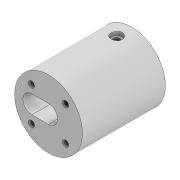
# Autodesk Inventor part: Part1_b_nmew
Saved by Autodesk Inventor 2021 (Build 250183000, 183)
## iProperties
Created: 2022-05-23
Part Number: Part1_b_nmew
Material: Generic
Document SubType Name: Modeling
Designer: romanp
Density: 1 g/cm^3
Appearance: Default
Author: romanp
Autodesk Inventor part; units mm, degrees
ref_plane "YZ Plane" through (0, 0, 0) normal (1, 0, 0) x (0, 1, 0)
ref_plane "XZ Plane" through (0, 0, 0) normal (0, 1, 0) x (-1, 0, 0)
ref_plane "XY Plane" through (0, 0, 0) normal (0, 0, 1) x (1, 0, 0)
sketch "Sketch11" plane through (0, 0, 0) normal (0, 0, 1) x (1, 0, 0)
  line L0 (-3.4593, 3.4593) -> (0, 0)
  line L1 (-3.4593, 3.4593) -> (-3.4593, 46.5407)
  line L2 (0, 50) -> (-3.4593, 46.5407)
  line L3 (43.0814, 50) -> (0, 50)
  line L4 (46.5407, 46.5407) -> (43.0814, 50)
  line L5 (46.5407, 3.4593) -> (46.5407, 46.5407)
  line L6 (43.0814, 0) -> (46.5407, 3.4593)
  line L7 (43.0814, 0) -> (0, 0)
  constraints: 16 end point
extrude "Extrusion8" add sketch "Sketch11" along normal blind 5
sketch "Sketch16" plane through (0, 0, 0) normal (0, 0, -1) x (-1, 0, 0)
  line L0 (-27.0407, 40) -> (-34.0407, 40)
  line L1 (-36.5407, 37.5) -> (-36.5407, 30.5)
  arc A0 (-34.0407, 40) -> (-36.5407, 37.5) centre (-34.0407, 37.5) ccw
  line L2 (-9.0407, 40) -> (-16.0407, 40)
  arc A1 (-6.5407, 37.5) -> (-9.0407, 40) centre (-9.0407, 37.5) ccw
  line L3 (-6.5407, 30.5) -> (-6.5407, 37.5)
  line L4 (-6.5407, 12.5) -> (-6.5407, 19.5)
  arc A2 (-9.0407, 10) -> (-6.5407, 12.5) centre (-9.0407, 12.5) ccw
  line L5 (-16.0407, 10) -> (-9.0407, 10)
  line L6 (-34.0407, 10) -> (-27.0407, 10)
  arc A3 (-36.5407, 12.5) -> (-34.0407, 10) centre (-34.0407, 12.5) ccw
  line L7 (-36.5407, 19.5) -> (-36.5407, 12.5)
  line L8 (0, 50) -> (3.4593, 46.5407) projected
  line L9 (-43.0814, 0) -> (-46.5407, 3.4593) projected
  line L10 (-46.5407, 46.5407) -> (-43.0814, 50) projected
  line L11 (-43.0814, 0) -> (-43.0814, 50)
  line L12 (3.4593, 3.4593) -> (0, 0) projected
  line L13 (-6.5407, 30.5) -> (-6.5407, 19.5)
  line L14 (-16.0407, 40) -> (-27.0407, 40)
  line L15 (-36.5407, 30.5) -> (-36.5407, 19.5)
  line L16 (-27.0407, 10) -> (-16.0407, 10)
  circle A4 centre (-2.5407, 44) radius 2.5
  circle A5 centre (-40.5407, 6) radius 2.5
  circle A6 centre (-2.5407, 6) radius 2.5
  circle A7 centre (-40.5407, 44) radius 2.5
  line L17 (0, 50) -> (3.4593, 46.5407)
  line L18 (3.4593, 46.5407) -> (3.4593, 3.4593) projected
  line L19 (0, 0) -> (-43.0814, 0) projected
  line L20 (3.4593, 3.4593) -> (0, 0)
  line L21 (0, 0) -> (-43.0814, 0)
  line L22 (-43.0814, 0) -> (-46.5407, 3.4593) projected
  line L23 (-43.0814, 0) -> (-46.5407, 3.4593)
  line L24 (-46.5407, 3.4593) -> (-46.5407, 46.5407) projected
  line L25 (-46.5407, 3.4593) -> (-46.5407, 46.5407)
  line L26 (-46.5407, 46.5407) -> (-43.0814, 50)
  line L27 (0, 50) -> (-43.0814, 50) projected
  line L28 (0, 50) -> (-43.0814, 50)
  dimension "d44" = 5
  dimension "d45" = 5
  dimension "d46" = 5
  dimension "d47" = 5
  constraints: 40 end point, 8 centre point, 8 collinear, 8 point on circle, 2 vertical, 1 perpendicular, 1 point on line
  measures "d44" diameter of A4
  measures "d45" diameter of A5
  measures "d46" diameter of A6
  measures "d47" diameter of A7
extrude "Extrusion11" add sketch "Sketch16" along normal blind 15
sketch "Sketch18" plane through (0, 0, -15) normal (0, 0, -1) x (-1, 0, 0)
  circle A0 centre (-2.5407, 6) radius 2.5 projected
  circle A1 centre (-2.5407, 6) radius 2.5
  circle A2 centre (-40.5407, 6) radius 2.5 projected
  circle A3 centre (-40.5407, 6) radius 2.5
  circle A4 centre (-40.5407, 44) radius 2.5 projected
  circle A5 centre (-40.5407, 44) radius 2.5
  circle A6 centre (-2.5407, 44) radius 2.5 projected
  circle A7 centre (-2.5407, 44) radius 2.5
  point P0 (0, 0)
  constraints: 4 centre point, 4 coincident
extrude "Extrusion12" cut sketch "Sketch18" against normal blind 100
sketch "Sketch19" plane through (0, 0, -15) normal (0, 0, -1) x (-1, 0, 0)
  circle A0 centre (-2.5407, 6) radius 2.5 projected
  circle A1 centre (-2.5407, 6) radius 4.3
  circle A2 centre (-40.5407, 6) radius 2.5 projected
  circle A3 centre (-40.5407, 6) radius 4.3
  circle A4 centre (-2.5407, 44) radius 2.5 projected
  circle A5 centre (-2.5407, 44) radius 4.3
  circle A6 centre (-40.5407, 44) radius 2.5 projected
  circle A7 centre (-40.5407, 44) radius 4.3
  point P0 (0, 0)
  dimension "d54" = 8.6
  dimension "d55" = 8.6
  dimension "d56" = 8.6
  dimension "d57" = 8.6
  constraints: 4 centre point, 4 coincident
  measures "d54" diameter of A1
  measures "d55" diameter of A3
  measures "d56" diameter of A5
  measures "d57" diameter of A7
extrude "Extrusion13" cut sketch "Sketch19" against normal blind 10 contours A0 | A1 | A2 | A3 | A5 | A6 | A7
sketch "Sketch20" plane through (0, 0, -15) normal (0, 0, -1) x (-1, 0, 0)
  line L0 (0, 50) -> (-43.0814, 50) projected
  line L1 (-43.0814, 50) -> (-46.5407, 46.5407) projected
  line L2 (-46.5407, 46.5407) -> (-46.5407, 3.4593) projected
  line L3 (-46.5407, 3.4593) -> (-43.0814, 0) projected
  line L4 (-43.0814, 0) -> (0, 0) projected
  line L5 (0, 0) -> (3.4593, 3.4593) projected
  line L6 (3.4593, 3.4593) -> (3.4593, 46.5407) projected
  line L7 (3.4593, 46.5407) -> (0, 50) projected
  circle A0 centre (-2.5407, 44) radius 4.3 projected
  circle A1 centre (-40.5407, 44) radius 4.3 projected
  circle A2 centre (-40.5407, 6) radius 4.3 projected
  circle A3 centre (-2.5407, 6) radius 4.3 projected
  arc A4 (-9.0407, 10) -> (-6.5407, 12.5) centre (-9.0407, 12.5) ccw projected
  line L8 (-9.0407, 10) -> (-34.0407, 10) projected
  line L9 (-36.5407, 12.5) -> (-36.5407, 37.5) projected
  arc A5 (-36.5407, 12.5) -> (-34.0407, 10) centre (-34.0407, 12.5) ccw projected
  line L10 (-6.5407, 37.5) -> (-6.5407, 12.5) projected
  arc A6 (-6.5407, 37.5) -> (-9.0407, 40) centre (-9.0407, 37.5) ccw projected
  line L11 (-34.0407, 40) -> (-9.0407, 40) projected
  arc A7 (-34.0407, 40) -> (-36.5407, 37.5) centre (-34.0407, 37.5) ccw projected
extrude "Extrusion14" add sketch "Sketch20" along normal blind 25
sketch "Sketch21" plane through (0, 50, 5) normal (0, 1, 0) x (1, 0, 0)
  line L0 (-1.7593, 45) -> (6.8407, 45) projected
  circle A0 centre (21.6907, 35) radius 2
  dimension "d63" = 4
  constraints: 1 centre point
  measures "d63" diameter of A0
extrude "Extrusion15" cut sketch "Sketch21" against normal blind 500
sketch "Sketch22" plane through (0, 50, 5) normal (0, 1, 0) x (1, 0, 0)
  circle A0 centre (21.6907, 35) radius 2 projected
  circle A1 centre (21.6907, 35) radius 3.75
  point P0 (0, 5)
  dimension "d67" = 7.5
  constraints: 1 centre point, 1 coincident
  measures "d67" diameter of A1
extrude "Extrusion16" cut sketch "Sketch22" against normal blind 5 contours A0 | A1
sketch "Sketch23" plane through (0, 0, 5) normal (0, -1, 0) x (1, 0, 0)
  circle A0 centre (21.6907, -35) radius 2 projected
  circle A1 centre (21.6907, -35) radius 3.75
  point P0 (0, -5)
  dimension "d70" = 7.5
  constraints: 1 centre point, 1 coincident
  measures "d70" diameter of A1
extrude "Extrusion17" cut sketch "Sketch23" against normal blind 5
sketch "Sketch25" plane through (0, 0, 5) normal (0, 0, 1) x (1, 0, 0)
  circle A0 centre (2.5407, 6) radius 2.5 projected
  circle A1 centre (40.5407, 44) radius 2.5 projected
  circle A2 centre (2.5407, 44) radius 2.5 projected
  circle A3 centre (40.5407, 6) radius 4.3 projected
  circle A4 centre (21.5407, 25) radius 9
  point P0 (0, 0)
  dimension "d75" = 18
  constraints: 1 centre point
  measures "d75" diameter of A4
extrude "Extrusion18" cut sketch "Sketch25" against normal blind 20 contours A4
sketch "Sketch27" plane through (0, 0, -40) normal (0, 0, -1) x (-1, 0, 0)
  circle A0 centre (-21.5407, 25) radius 10
  circle A1 centre (-21.5407, 25) radius 9 projected
  circle A2 centre (-21.5407, 25) radius 22.5
  circle A3 centre (-21.5407, 25) radius 40.9487
  point P0 (0, 0)
  dimension "d78" = 45
  constraints: 3 centre point, 2 coincident
  measures "d78" diameter of A2
extrude "Extrusion19" cut sketch "Sketch27" against normal blind 100 contours A3
sketch "Sketch28" plane through (21.5407, 25, -40) normal (0, 0, -1) x (-1, 0, 0)
  circle A0 centre (0, 0) radius 10
  circle A1 centre (-11.3137, -11.3137) radius 4.5
  circle A2 centre (-11.3137, 11.3137) radius 4.5
  circle A3 centre (11.3137, 11.3137) radius 4.5
  circle A4 centre (11.3137, -11.3137) radius 4.5
  point P0 (21.5407, -25)
  dimension "d81" = 9
  dimension "d82" = 9
  dimension "d83" = 9
  dimension "d84" = 9
  constraints: 5 centre point
  measures "d81" diameter of A1
  measures "d82" diameter of A2
  measures "d83" diameter of A3
  measures "d84" diameter of A4
extrude "Extrusion20" cut sketch "Sketch28" against normal blind 100 contours A1 | A2 | A3 | A4
sketch "Sketch29" plane through (21.5407, 25, 5) normal (0, 0, 1) x (1, 0, 0)
  circle A0 centre (0, 0) radius 22.5 projected
  circle A1 centre (-11.3137, 11.3137) radius 4.5 projected
  circle A2 centre (-11.3137, -11.3137) radius 4.5 projected
  circle A3 centre (11.3137, -11.3137) radius 4.5 projected
  circle A4 centre (11.3137, 11.3137) radius 4.5 projected
  circle A5 centre (0, 0) radius 9 projected
  circle A6 centre (-11.3137, -11.3137) radius 2
  circle A7 centre (-11.3137, 11.3137) radius 2
  circle A8 centre (11.3137, 11.3137) radius 2
  circle A9 centre (11.3137, -11.3137) radius 2
  point P0 (-21.5407, -25)
  dimension "d87" = 4
  dimension "d88" = 4
  dimension "d89" = 4
  dimension "d90" = 4
  constraints: 4 centre point, 4 coincident
  measures "d87" diameter of A6
  measures "d88" diameter of A7
  measures "d89" diameter of A8
  measures "d90" diameter of A9
extrude "Extrusion21" add sketch "Sketch29" along normal blind 10 contours A0 | A1 | A2 | A3 | A4
sketch "Sketch32" plane through (21.5407, 25, -40) normal (0, 0, -1) x (-1, 0, 0)
  circle A0 centre (0, 0) radius 9 projected
  line L0 (0, 0) -> (0, 15.25)
  line L1 (0, 15.25) -> (-15.25, 15.25)
  line L2 (0, 0) -> (0, -15.25)
  line L3 (0, -15.25) -> (15.25, -15.25)
  line L4 (-15.25, 15.25) -> (15.25, 15.25)
  line L5 (15.25, 15.25) -> (15.25, -15.25)
  line L6 (15.25, -15.25) -> (-15.25, -15.25)
  line L7 (-15.25, -15.25) -> (-15.25, 15.25)
  arc A1 (-8.7328, 15) -> (-15, 8.7328) centre (-11.3137, 11.3137) ccw projected
  line L8 (-8.7328, 15) -> (8.7328, 15) projected
  arc A2 (15, 8.7328) -> (8.7328, 15) centre (11.3137, 11.3137) ccw projected
  line L9 (15, 8.7328) -> (15, -8.7328) projected
  arc A3 (8.7328, -15) -> (15, -8.7328) centre (11.3137, -11.3137) ccw projected
  line L10 (8.7328, -15) -> (-8.7328, -15) projected
  arc A4 (-15, -8.7328) -> (-8.7328, -15) centre (-11.3137, -11.3137) ccw projected
  line L11 (-15, -8.7328) -> (-15, 8.7328) projected
  circle A5 centre (0, 0) radius 22.5 projected
  point P0 (21.5407, -25)
  point P1 (-9.133, -15.25)
  point P2 (9.133, -15.25)
  point P3 (15.25, -9.133)
  point P4 (15.25, 9.133)
  point P5 (9.133, 15.25)
  point P6 (0, 15.25)
  point P7 (-9.133, 15.25)
  point P8 (-15.25, 9.133)
  point P9 (-15.25, -9.133)
  dimension "d93" = 15.25
  dimension "d94" = 15.25
  dimension "d95" = 15.25
  dimension "d96" = 15.25
  constraints: 16 end point, 3 perpendicular, 2 parallel, 2 vertical, 1 horizontal
  measures "d93" distance of L0.start L0.end
  measures "d94" distance of L0.end L1.end
  measures "d95" distance of L0.start L2.end
  measures "d96" distance of L2.end L3.end
extrude "Extrusion22" cut sketch "Sketch32" against normal blind 40 contours L8 A1 L1 L0 | L0 L4 A2 L8 | L10 A3 L3 L2 | L2 L6 A4 L10 | A1 L11 A4 L7 | L5 A3 L9 A2
sketch "Sketch33" plane through (10.227, 36.3137, 5) normal (0, 0, -1) x (-1, 0, 0)
  circle A0 centre (0, 0) radius 2 projected
  circle A1 centre (0, 0) radius 4.5 projected
  circle A2 centre (-22.6274, 0) radius 2 projected
  circle A3 centre (-22.6274, 0) radius 4.5 projected
  circle A4 centre (-22.6274, -22.6274) radius 2 projected
  circle A5 centre (-22.6274, -22.6274) radius 4.5 projected
  circle A6 centre (0, -22.6274) radius 2 projected
  circle A7 centre (0, -22.6274) radius 4.5 projected
  point P0 (10.227, -36.3137)
extrude "Extrusion23" add sketch "Sketch33" along normal blind 2
sketch "Sketch34" plane through (0, 0, 0) normal (0, 0, -1) x (-1, 0, 0)
  circle A0 centre (-21.5407, 25) radius 9 projected
  arc A1 (-36.7907, 34.133) -> (-30.6737, 40.25) centre (-32.8544, 36.3137) ccw projected
  line L0 (-36.7907, 15.867) -> (-36.7907, 34.133) projected
  arc A2 (-30.6737, 9.75) -> (-36.7907, 15.867) centre (-32.8544, 13.6863) ccw projected
  line L1 (-12.4077, 9.75) -> (-30.6737, 9.75) projected
  arc A3 (-6.2907, 15.867) -> (-12.4077, 9.75) centre (-10.227, 13.6863) ccw projected
  line L2 (-6.2907, 34.133) -> (-6.2907, 15.867) projected
  arc A4 (-12.4077, 40.25) -> (-6.2907, 34.133) centre (-10.227, 36.3137) ccw projected
  line L3 (-30.6737, 40.25) -> (-12.4077, 40.25) projected
  point P0 (0, 0)
extrude "Extrusion24" add sketch "Sketch34" along normal blind 2
sketch "Sketch35" plane through (0, 0, -2) normal (0, 0, -1) x (-1, 0, 0)
  circle A0 centre (-10.227, 36.3137) radius 2 projected
  line L0 (-10.227, 25.0002) -> (-32.8544, 25.0002)
  circle A1 centre (-10.227, 25.0002) radius 6
  circle A2 centre (-32.8544, 25.0002) radius 6
  point P0 (0, 0)
  dimension "d103" = 11.3135
  dimension "d104" = 12
  dimension "d105" = 12
  constraints: 2 centre point, 2 coincident, 2 end point
  measures "d103" distance of A0.centre L0.start
  measures "d104" diameter of A1
  measures "d105" diameter of A2
extrude "Extrusion25" cut sketch "Sketch35" along normal mid plane 100 contours A1 | A2
sketch "Sketch36" plane through (0, 0, -2) normal (0, 0, -1) x (-1, 0, 0)
  arc A0 (-29.1862, 29.7483) -> (-29.1864, 20.252) centre (-32.8544, 25.0002) ccw projected
  line L0 (-32.8544, 25.0002) -> (-32.8544, 31.0002)
  arc A1 (-13.895, 20.252) -> (-13.8952, 29.7483) centre (-10.227, 25.0002) ccw projected
  line L1 (-10.227, 25.0002) -> (-10.227, 31.0002)
  line L2 (-10.227, 31.0002) -> (-32.8544, 31.0002)
  line L3 (-10.227, 25.0002) -> (-10.227, 19.0002)
  line L4 (-32.8544, 25.0002) -> (-32.8544, 19.0002)
  line L5 (-32.8544, 19.0002) -> (-10.227, 19.0002)
  arc A2 (-29.1862, 29.7483) -> (-36.7907, 29.5285) centre (-32.8544, 25.0002) ccw projected
  arc A3 (-13.8952, 29.7483) -> (-29.1862, 29.7483) centre (-21.5407, 25) ccw projected
  arc A4 (-6.2907, 29.5285) -> (-13.8952, 29.7483) centre (-10.227, 25.0002) ccw projected
  line L6 (-6.2907, 34.133) -> (-6.2907, 29.5285) projected
  arc A5 (-12.4077, 40.25) -> (-6.2907, 34.133) centre (-10.227, 36.3137) ccw projected
  line L7 (-30.6737, 40.25) -> (-12.4077, 40.25) projected
  arc A6 (-36.7907, 34.133) -> (-30.6737, 40.25) centre (-32.8544, 36.3137) ccw projected
  line L8 (-36.7907, 29.5285) -> (-36.7907, 34.133) projected
  arc A7 (-36.7907, 20.4719) -> (-29.1864, 20.252) centre (-32.8544, 25.0002) ccw projected
  line L9 (-36.7907, 15.867) -> (-36.7907, 20.4719) projected
  arc A8 (-30.6737, 9.75) -> (-36.7907, 15.867) centre (-32.8544, 13.6863) ccw projected
  line L10 (-12.4077, 9.75) -> (-30.6737, 9.75) projected
  arc A9 (-6.2907, 15.867) -> (-12.4077, 9.75) centre (-10.227, 13.6863) ccw projected
  line L11 (-6.2907, 20.4719) -> (-6.2907, 15.867) projected
  arc A10 (-13.895, 20.252) -> (-6.2907, 20.4719) centre (-10.227, 25.0002) ccw projected
  arc A11 (-29.1864, 20.252) -> (-13.895, 20.252) centre (-21.5407, 25) ccw projected
  point P0 (0, 0)
  point P1 (-28.2491, 19.0002)
  point P2 (-28.2487, 31.0002)
  point P3 (-14.8323, 19.0002)
  point P4 (-14.8327, 31.0002)
  point P5 (-13.8952, 29.7483)
  constraints: 12 end point, 3 point on circle, 2 perpendicular, 2 tangent, 2 vertical, 1 point on line
extrude "Extrusion26" cut sketch "Sketch36" against normal blind 100 contours A0 L2 A3 | L2 A1 A3 | A0 A11 L5 | A11 A1 L5
sketch "Sketch37" plane through (0, 0, -2) normal (0, 0, -1) x (-1, 0, 0)
  arc A0 (-36.7907, 20.4719) -> (-32.8544, 19.0002) centre (-32.8544, 25.0002) ccw projected
  line L0 (-32.8544, 25.0002) -> (-32.8544, 31.0002)
  arc A1 (-6.2907, 29.5285) -> (-10.227, 31.0002) centre (-10.227, 25.0002) ccw projected
  line L1 (-32.8544, 31.0002) -> (-10.227, 31.0002)
  arc A2 (-10.227, 19.0002) -> (-10.227, 31.0002) centre (-10.227, 25.0002) ccw projected
  line L2 (-10.227, 31.0002) -> (-10.227, 19.0002)
  line L3 (-10.227, 19.0002) -> (-32.8544, 19.0002)
  line L4 (-32.8544, 19.0002) -> (-32.8544, 25.0002)
  line L5 (-32.8544, 31.0002) -> (-28.2487, 31.0002) projected
  arc A3 (-14.8327, 31.0002) -> (-28.2487, 31.0002) centre (-21.5407, 25) ccw projected
  line L6 (-14.8327, 31.0002) -> (-10.227, 31.0002) projected
  arc A4 (-6.2907, 29.5285) -> (-10.227, 31.0002) centre (-10.227, 25.0002) ccw projected
  line L7 (-6.2907, 34.133) -> (-6.2907, 29.5285) projected
  arc A5 (-12.4077, 40.25) -> (-6.2907, 34.133) centre (-10.227, 36.3137) ccw projected
  line L8 (-30.6737, 40.25) -> (-12.4077, 40.25) projected
  arc A6 (-36.7907, 34.133) -> (-30.6737, 40.25) centre (-32.8544, 36.3137) ccw projected
  line L9 (-36.7907, 29.5285) -> (-36.7907, 34.133) projected
  arc A7 (-32.8544, 31.0002) -> (-36.7907, 29.5285) centre (-32.8544, 25.0002) ccw projected
  line L10 (-10.227, 19.0002) -> (-14.8323, 19.0002) projected
  arc A8 (-28.2491, 19.0002) -> (-14.8323, 19.0002) centre (-21.5407, 25) ccw projected
  line L11 (-28.2491, 19.0002) -> (-32.8544, 19.0002) projected
  arc A9 (-36.7907, 20.4719) -> (-32.8544, 19.0002) centre (-32.8544, 25.0002) ccw projected
  line L12 (-36.7907, 15.867) -> (-36.7907, 20.4719) projected
  arc A10 (-30.6737, 9.75) -> (-36.7907, 15.867) centre (-32.8544, 13.6863) ccw projected
  line L13 (-12.4077, 9.75) -> (-30.6737, 9.75) projected
  arc A11 (-6.2907, 15.867) -> (-12.4077, 9.75) centre (-10.227, 13.6863) ccw projected
  line L14 (-6.2907, 20.4719) -> (-6.2907, 15.867) projected
  arc A12 (-10.227, 19.0002) -> (-6.2907, 20.4719) centre (-10.227, 25.0002) ccw projected
  point P0 (0, 0)
  point P1 (-28.2491, 19.0002)
  constraints: 10 end point, 3 perpendicular, 2 tangent, 1 collinear, 1 point on line, 1 vertical
extrude "Extrusion27" add sketch "Sketch37" against normal blind 17 contours L3 A8 | A3 L1
sketch "Sketch38" plane through (0, 0, -2) normal (0, 0, -1) x (-1, 0, 0)
  arc A0 (-10.227, 19.0002) -> (-6.2907, 20.4719) centre (-10.227, 25.0002) ccw projected
  circle A1 centre (-10.227, 25.0002) radius 6
  line L0 (-32.8544, 31.0002) -> (-10.227, 31.0002) projected
  arc A2 (-6.2907, 29.5285) -> (-10.227, 31.0002) centre (-10.227, 25.0002) ccw projected
  line L1 (-6.2907, 34.133) -> (-6.2907, 29.5285) projected
  arc A3 (-12.4077, 40.25) -> (-6.2907, 34.133) centre (-10.227, 36.3137) ccw projected
  line L2 (-30.6737, 40.25) -> (-12.4077, 40.25) projected
  arc A4 (-36.7907, 34.133) -> (-30.6737, 40.25) centre (-32.8544, 36.3137) ccw projected
  line L3 (-36.7907, 29.5285) -> (-36.7907, 34.133) projected
  arc A5 (-32.8544, 31.0002) -> (-36.7907, 29.5285) centre (-32.8544, 25.0002) ccw projected
  line L4 (-10.227, 19.0002) -> (-32.8544, 19.0002) projected
  arc A6 (-36.7907, 20.4719) -> (-32.8544, 19.0002) centre (-32.8544, 25.0002) ccw projected
  line L5 (-36.7907, 15.867) -> (-36.7907, 20.4719) projected
  arc A7 (-30.6737, 9.75) -> (-36.7907, 15.867) centre (-32.8544, 13.6863) ccw projected
  line L6 (-12.4077, 9.75) -> (-30.6737, 9.75) projected
  arc A8 (-6.2907, 15.867) -> (-12.4077, 9.75) centre (-10.227, 13.6863) ccw projected
  line L7 (-6.2907, 20.4719) -> (-6.2907, 15.867) projected
  arc A9 (-10.227, 19.0002) -> (-6.2907, 20.4719) centre (-10.227, 25.0002) ccw projected
  arc A10 (-36.7907, 29.5285) -> (-36.7907, 20.4719) centre (-32.8544, 25.0002) ccw projected
  line L8 (-36.7907, 29.5285) -> (-36.7907, 34.133) projected
  arc A11 (-30.6737, 40.25) -> (-36.7907, 34.133) centre (-32.8544, 36.3137) ccw projected
  line L9 (-30.6737, 40.25) -> (-12.4077, 40.25) projected
  arc A12 (-6.2907, 34.133) -> (-12.4077, 40.25) centre (-10.227, 36.3137) ccw projected
  line L10 (-6.2907, 34.133) -> (-6.2907, 29.5285) projected
  arc A13 (-6.2907, 20.4719) -> (-6.2907, 29.5285) centre (-10.227, 25.0002) ccw projected
  line L11 (-6.2907, 20.4719) -> (-6.2907, 15.867) projected
  arc A14 (-12.4077, 9.75) -> (-6.2907, 15.867) centre (-10.227, 13.6863) ccw projected
  line L12 (-12.4077, 9.75) -> (-30.6737, 9.75) projected
  arc A15 (-36.7907, 15.867) -> (-30.6737, 9.75) centre (-32.8544, 13.6863) ccw projected
  line L13 (-36.7907, 15.867) -> (-36.7907, 20.4719) projected
  circle A16 centre (-21.5407, 25) radius 22.5 projected
  point P0 (0, 0)
  point P1 (-10.227, 19.0002)
  constraints: 1 centre point, 1 coincident
extrude "Extrusion28" add sketch "Sketch38" against normal blind 17 contours L4 A6 A10 A5 L0 A1
sketch "Sketch39" plane through (0, 0, -2) normal (0, 0, -1) x (-1, 0, 0)
  arc A0 (-6.2907, 29.5285) -> (-6.2907, 20.4719) centre (-10.227, 25.0002) ccw projected
  line L0 (-6.2907, 34.133) -> (-6.2907, 29.5285) projected
  arc A1 (-12.4077, 40.25) -> (-6.2907, 34.133) centre (-10.227, 36.3137) ccw projected
  line L1 (-30.6737, 40.25) -> (-12.4077, 40.25) projected
  arc A2 (-36.7907, 34.133) -> (-30.6737, 40.25) centre (-32.8544, 36.3137) ccw projected
  line L2 (-36.7907, 29.5285) -> (-36.7907, 34.133) projected
  arc A3 (-36.7907, 29.5285) -> (-36.7907, 20.4719) centre (-32.8544, 25.0002) ccw projected
  line L3 (-36.7907, 15.867) -> (-36.7907, 20.4719) projected
  arc A4 (-30.6737, 9.75) -> (-36.7907, 15.867) centre (-32.8544, 13.6863) ccw projected
  line L4 (-12.4077, 9.75) -> (-30.6737, 9.75) projected
  arc A5 (-6.2907, 15.867) -> (-12.4077, 9.75) centre (-10.227, 13.6863) ccw projected
  line L5 (-6.2907, 20.4719) -> (-6.2907, 15.867) projected
  arc A6 (-36.7907, 29.5285) -> (-36.7907, 20.4719) centre (-32.8544, 25.0002) ccw projected
  line L6 (-36.7907, 20.4719) -> (-36.7907, 29.5285)
  point P0 (0, 0)
  constraints: 2 end point, 1 vertical
extrude "Extrusion29" add sketch "Sketch39" along normal blind 38 contours L6 A3
sketch "Sketch42" plane through (0, 0, -2) normal (0, 0, -1) x (-1, 0, 0)
  arc A0 (-6.2907, 29.5285) -> (-6.2907, 20.4719) centre (-10.227, 25.0002) ccw projected
  circle A1 centre (-10.227, 25.0002) radius 6
  point P0 (0, 0)
  point P1 (-6.2907, 20.4719)
  point P2 (-6.2907, 29.5285)
  constraints: 1 centre point, 1 coincident
extrude "Extrusion31" add sketch "Sketch42" against normal blind 17
sketch "Sketch43" plane through (10.227, 36.3137, 3) normal (0, 0, -1) x (-1, 0, 0)
  circle A0 centre (0, 0) radius 2 projected
  line L0 (0, 0) -> (0, -11.314)
  line L1 (0, -11.314) -> (-0.314, -11.314)
  circle A1 centre (-0.314, -11.314) radius 6
  point P0 (10.227, -36.3137)
  dimension "d121" = 11.314
  dimension "d122" = 0.314
  dimension "d123" = 12
  constraints: 4 end point, 1 centre point, 1 coincident, 1 horizontal, 1 vertical
  measures "d121" distance of L0.start L0.end
  measures "d122" distance of L0.end L1.end
  measures "d123" diameter of A1
extrude "Extrusion32" cut sketch "Sketch43" against normal mid plane 100 contours A1
sketch "Sketch44" plane through (0, 0, -2) normal (0, 0, -1) x (-1, 0, 0)
  circle A0 centre (-10.541, 24.9997) radius 6 projected
  arc A1 (-6.2907, 20.4719) -> (-6.2907, 29.5285) centre (-10.227, 25.0002) ccw projected
  circle A2 centre (-10.541, 24.9997) radius 6.2109
  line L0 (-6.2907, 20.4719) -> (-6.2907, 15.867) projected
  line L1 (-6.2907, 20.4719) -> (-6.2907, 29.5285)
  point P0 (0, 0)
  point P1 (-6.2907, 20.7647)
  point P2 (-6.2907, 29.2347)
  constraints: 2 end point, 1 coincident, 1 collinear, 3 other
extrude "Extrusion33" add sketch "Sketch44" along normal blind 38 contours A0 L1 A2 | A1 A2 picked at (-5.7662, 28.7111)
sketch "Sketch45" plane through (0, 0, -2) normal (0, 0, -1) x (-1, 0, 0)
  line L0 (-6.2907, 20.7647) -> (-6.2907, 15.867) projected
  arc A0 (-6.2907, 29.2347) -> (-6.2907, 20.7647) centre (-10.541, 24.9997) ccw projected
  line L1 (-6.2907, 34.133) -> (-6.2907, 29.2347) projected
  arc A1 (-12.4077, 40.25) -> (-6.2907, 34.133) centre (-10.227, 36.3137) ccw projected
  line L2 (-30.6737, 40.25) -> (-12.4077, 40.25) projected
  arc A2 (-36.7907, 34.133) -> (-30.6737, 40.25) centre (-32.8544, 36.3137) ccw projected
  line L3 (-36.7907, 15.867) -> (-36.7907, 34.133) projected
  arc A3 (-30.6737, 9.75) -> (-36.7907, 15.867) centre (-32.8544, 13.6863) ccw projected
  line L4 (-12.4077, 9.75) -> (-30.6737, 9.75) projected
  arc A4 (-6.2907, 15.867) -> (-12.4077, 9.75) centre (-10.227, 13.6863) ccw projected
  point P0 (0, 0)
extrude "Extrusion34" add sketch "Sketch45" along normal blind 14.2
sketch "Sketch46" plane through (0, 0, -16.2) normal (0, 0, -1) x (-1, 0, 0)
  circle A0 centre (-32.8544, 13.6863) radius 2 projected
  circle A1 centre (-10.227, 36.3137) radius 2 projected
  circle A2 centre (-32.8544, 36.3137) radius 2 projected
  circle A3 centre (-10.227, 13.6863) radius 2 projected
  circle A4 centre (-21.5407, 25) radius 6
  line L0 (-21.5407, 25) -> (-21.5407, 31)
  line L1 (-21.5407, 31) -> (-10.5408, 30.9997)
  circle A5 centre (-10.541, 24.9997) radius 6 projected
  line L2 (-21.5407, 19) -> (-10.5412, 18.9997)
  point P0 (0, 0)
  dimension "d130" = 12
  constraints: 6 end point, 4 point on circle, 2 tangent, 1 centre point, 1 point on line, 1 vertical
  measures "d130" diameter of A4
extrude "Extrusion35" cut sketch "Sketch46" against normal blind 100 contours A4 A5 | L1 A5 A4 | A4 A5 L2 picked at (-23.845, 25)
sketch "Sketch47" plane through (21.5407, 25, -40) normal (0, 0, -1) x (-1, 0, 0)
  line L0 (-15.25, -9.133) -> (-15.25, 9.133) projected
  arc A0 (-9.133, 15.25) -> (-15.25, 9.133) centre (-11.3137, 11.3137) ccw projected
  line L1 (-9.133, 15.25) -> (9.133, 15.25) projected
  arc A1 (15.25, 9.133) -> (9.133, 15.25) centre (11.3137, 11.3137) ccw projected
  line L2 (15.25, 9.133) -> (15.25, 4.2347) projected
  arc A2 (15.25, -4.2353) -> (15.25, 4.2347) centre (10.9997, -0.0003) ccw projected
  line L3 (15.25, -4.2353) -> (15.25, -9.133) projected
  arc A3 (9.133, -15.25) -> (15.25, -9.133) centre (11.3137, -11.3137) ccw projected
  line L4 (9.133, -15.25) -> (-9.133, -15.25) projected
  arc A4 (-15.25, -9.133) -> (-9.133, -15.25) centre (-11.3137, -11.3137) ccw projected
  circle A5 centre (0, 0) radius 22.5 projected
  line L5 (10.9995, -6.0003) -> (0, -6) projected
  arc A6 (0, 6) -> (0, -6) centre (0, 0) ccw projected
  line L6 (0, 6) -> (10.9999, 5.9997) projected
  arc A7 (15.25, 4.2347) -> (10.9999, 5.9997) centre (10.9997, -0.0003) ccw projected
  line L7 (15.25, 9.133) -> (15.25, 4.2347) projected
  arc A8 (9.133, 15.25) -> (15.25, 9.133) centre (11.3137, 11.3137) ccw projected
  line L8 (-9.133, 15.25) -> (9.133, 15.25) projected
  arc A9 (-15.25, 9.133) -> (-9.133, 15.25) centre (-11.3137, 11.3137) ccw projected
  line L9 (-15.25, -9.133) -> (-15.25, 9.133) projected
  arc A10 (-9.133, -15.25) -> (-15.25, -9.133) centre (-11.3137, -11.3137) ccw projected
  line L10 (9.133, -15.25) -> (-9.133, -15.25) projected
  arc A11 (15.25, -9.133) -> (9.133, -15.25) centre (11.3137, -11.3137) ccw projected
  line L11 (15.25, -4.2353) -> (15.25, -9.133) projected
  arc A12 (10.9995, -6.0003) -> (15.25, -4.2353) centre (10.9997, -0.0003) ccw projected
  arc A13 (-15.1, -9.0052) -> (-9.0052, -15.1) centre (-11.1369, -11.1369) ccw
  line L12 (-15.1, -9.0052) -> (-15.1, 9.0052)
  arc A14 (-9.0052, 15.1) -> (-15.1, 9.0052) centre (-11.1369, 11.1369) ccw
  line L13 (-9.0052, 15.1) -> (9.0052, 15.1)
  arc A15 (15.1, 9.0052) -> (9.0052, 15.1) centre (11.1369, 11.1369) ccw
  line L14 (15.1, 9.0052) -> (15.1, -9.0052)
  arc A16 (9.0052, -15.1) -> (15.1, -9.0052) centre (11.1369, -11.1369) ccw
  line L15 (9.0052, -15.1) -> (-9.0052, -15.1)
  point P0 (21.5407, -25)
  point P1 (-8.8818, 15.1)
  point P2 (8.8818, 15.1)
  point P3 (-15.1, -8.8818)
  point P4 (-15.1, 8.8818)
  point P5 (8.8818, -15.1)
  point P6 (-8.8818, -15.1)
  point P7 (15.1, -4.3807)
  point P8 (15.1, -8.8818)
  point P9 (15.1, 8.8818)
  point P10 (15.1, 4.3801)
  constraints: 8 end point, 8 point on circle, 4 centre point
extrude "Extrusion36" add sketch "Sketch47" against normal blind 23.8 contours L0 A9 L12 A10 | A10 L15 A11 L4 | L1 A8 L13 A9 | A11 L14 A12 L3 | L2 A7 L14 A8
sketch "Sketch48" plane through (21.6907, 5, -30) normal (0, -1, 0) x (1, 0, 0)
  circle A0 centre (0, 0) radius 2.05
  point P0 (-21.6907, 30)
  dimension "d135" = 4.1
  constraints: 1 centre point
  measures "d135" diameter of A0
extrude "Extrusion37" cut sketch "Sketch48" against normal blind 100
sketch "Sketch49" plane through (0, 0, -16.2) normal (0, 0, -1) x (-1, 0, 0)
  circle A0 centre (-32.8544, 36.3137) radius 2 projected
  circle A1 centre (-32.8544, 36.3137) radius 2.05
  circle A2 centre (-10.227, 36.3137) radius 2 projected
  circle A3 centre (-10.227, 36.3137) radius 2.05
  circle A4 centre (-32.8544, 13.6863) radius 2 projected
  circle A5 centre (-32.8544, 13.6863) radius 2.05
  circle A6 centre (-10.227, 13.6863) radius 2 projected
  circle A7 centre (-10.227, 13.6863) radius 2.05
  point P0 (0, 0)
  dimension "d138" = 4.1
  dimension "d139" = 4.1
  dimension "d140" = 4.1
  dimension "d141" = 4.1
  constraints: 4 centre point, 4 coincident
  measures "d138" diameter of A1
  measures "d139" diameter of A3
  measures "d140" diameter of A5
  measures "d141" diameter of A7
extrude "Extrusion38" cut sketch "Sketch49" against normal blind 100 contours A0 | A1 | A2 | A3 | A4 | A5 | A6 | A7
sketch "Sketch50" plane through (21.5407, 25, -40) normal (0, 0, -1) x (-1, 0, 0)
  arc A0 (-12.7512, 15.3015) -> (-15.3015, 12.7513) centre (-12.7512, 12.7513) ccw
  circle A1 centre (0, 0) radius 1
  line L0 (-15.3015, -12.7512) -> (-15.3015, 12.7513)
  line L1 (-12.7512, 15.3015) -> (12.7513, 15.3015)
  arc A2 (-15.3015, -12.7512) -> (-12.7513, -15.3015) centre (-12.7513, -12.7512) ccw
  arc A3 (15.3015, 12.7512) -> (12.7513, 15.3015) centre (12.7513, 12.7512) ccw
  line L2 (12.7512, -15.3015) -> (-12.7513, -15.3015)
  line L3 (15.3015, 12.7512) -> (15.3015, -12.7513)
  arc A4 (12.7512, -15.3015) -> (15.3015, -12.7513) centre (12.7512, -12.7513) ccw
  arc A5 (0, 6) -> (0, -6) centre (0, 0) ccw projected
  point P0 (21.5407, -25)
  dimension "d144" = 2
  constraints: 8 end point, 8 point on circle, 5 centre point
  measures "d144" diameter of A1
extrude "Extrusion39" cut sketch "Sketch50" against normal blind 23.8
sketch "Sketch51" plane through (21.5407, 25, -40) normal (0, 0, -1) x (-1, 0, 0)
  arc A0 (13.7471, -15.099) -> (15.099, -13.7471) centre (11.3137, -11.3137) ccw projected
  arc A1 (13.7471, -15.099) -> (15.099, -13.7471) centre (12.7512, -12.7513) ccw projected
  arc A2 (-15.099, -13.7471) -> (-13.7471, -15.099) centre (-11.3137, -11.3137) ccw projected
  arc A3 (-15.099, -13.7471) -> (-13.7471, -15.099) centre (-12.7513, -12.7512) ccw projected
  arc A4 (-13.7471, 15.099) -> (-15.099, 13.7471) centre (-11.3137, 11.3137) ccw projected
  arc A5 (-13.7471, 15.099) -> (-15.099, 13.7471) centre (-12.7512, 12.7513) ccw projected
  arc A6 (15.099, 13.7471) -> (13.7471, 15.099) centre (11.3137, 11.3137) ccw projected
  arc A7 (15.099, 13.7471) -> (13.7471, 15.099) centre (12.7513, 12.7512) ccw projected
  point P0 (21.5407, -25)
extrude "Extrusion40" cut sketch "Sketch51" against normal blind 43
body "Solid2"
